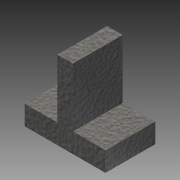
# Autodesk Inventor part: Part1
Saved by Autodesk Inventor 2014 SP2 (Build 180246200, 246)
## iProperties
Created: 2019-07-04
Part Number: Part1
Material: Generic
Document SubType Name: Modeling
Designer: USER PC
Density: 1 g/cm^3
Appearance: Steel - Cast
Mass: 2.07497 g
Surface Area: 13.5977 cm^2
Volume: 2.07497 cm^3
Author: USER PC
Autodesk Inventor part; units mm, degrees
ref_plane "YZ Plane" through (0, 0, 0) normal (1, 0, 0) x (0, 1, 0)
ref_plane "XZ Plane" through (0, 0, 0) normal (0, 1, 0) x (-1, 0, 0)
ref_plane "XY Plane" through (0, 0, 0) normal (0, 0, 1) x (1, 0, 0)
sketch "Sketch1" plane through (0, 0, 0) normal (0, 0, 1) x (1, 0, 0)
  line L0 (-10.3132, 5.9874) -> (10.3132, 5.9874)
  line L1 (10.3132, 5.9874) -> (10.3132, -6.7322)
  line L2 (10.3132, -6.7322) -> (-10.3132, -6.7322)
  line L3 (-10.3132, -6.7322) -> (-10.3132, 5.9874)
  line L4 (-10.3132, 5.9874) -> (10.3132, -6.7322) construction
  line L5 (10.3132, 5.9874) -> (-10.3132, -6.7322) construction
  point P0 (0, 0)
  point P1 (0, -0.3724)
  constraints: 12 end point, 2 midpoint, 2 parallel, 1 horizontal, 1 perpendicular
extrude "Extrusion1" add sketch "Sketch1" along normal blind 5
sketch "Sketch2" plane through (0, 0, 5) normal (0, 0, 1) x (1, 0, 0)
  line L0 (10.3132, 5.9874) -> (-10.3132, 5.9874) projected
  line L1 (-10.3132, -6.7322) -> (10.3132, -6.7322) projected
  line L2 (0, 5.9874) -> (2, 5.9874)
  line L3 (2, 5.9874) -> (2, -6.7322)
  line L4 (2, -6.7322) -> (-2, -6.7322)
  line L5 (-2, -6.7322) -> (-2, 5.9874)
  line L6 (0, 5.9874) -> (-2, 5.9874)
  dimension "d2" = 2
  dimension "d3" = 4
  constraints: 10 end point, 4 point on line, 3 perpendicular, 1 midpoint
  measures "d2" distance of L2.start L2.end
  measures "d3" distance of L3.end L4.end
extrude "Extrusion2" add sketch "Sketch2" along normal blind 15
body "Solid1"
